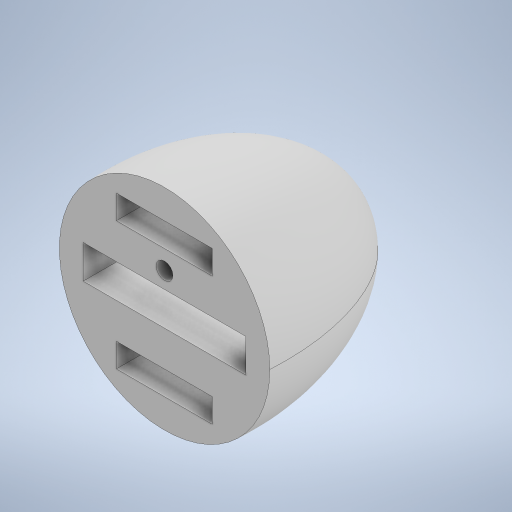
# Autodesk Inventor part: Bead Round Top copy 1
Saved by Autodesk Inventor 2024 (Build 280153000, 153)
## iProperties
Created: 2024-06-20
Part Number: Bead Round Top copy 1
Material: Generic
Document SubType Name: Modeling
Designer: waiy
Density: 1 g/cm^3
Appearance: Default
Author: waiy
Autodesk Inventor part; units mm, degrees
ref_plane "YZ Plane" through (0, 0, 0) normal (1, 0, 0) x (0, 1, 0)
ref_plane "XZ Plane" through (0, 0, 0) normal (0, 1, 0) x (-1, 0, 0)
ref_plane "XY Plane" through (0, 0, 0) normal (0, 0, 1) x (1, 0, 0)
sketch "Sketch1" plane through (0, 0, 0) normal (0, 1, 0) x (-1, 0, 0)
  ellipse E0 centre (0, 0) end of major axis (0, 17.78) minor radius 11.2075
  line L0 (11.1609, 1.6196) -> (-11.1609, 1.6196)
  line L1 (0, -17.78) -> (0, 1.6196)
  line L2 (8.595, 11.4106) -> (-8.6719, 11.4106)
  dimension "d0" = 17.78
  dimension "d11" = 9.7909
  constraints: 6 end point, 2 horizontal, 1 coincident, 1 midpoint, 6 other
  measures "d11" distance between parallel lines of L2 L0
revolve "Revolution1" add sketch "Sketch1" angle 360 about axis through (0, 0, -17.78) along (0, 0, 1) picked at (-2.3015, -10.0552) contours L0 L1 E0
sketch "Sketch2" plane through (0, 0, 1.6196) normal (0, 0, 1) x (1, 0, 0)
  line L0 (-8.636, 1.778) -> (8.636, 1.778)
  line L1 (8.636, 1.778) -> (8.636, -1.778)
  line L2 (8.636, -1.778) -> (-8.636, -1.778)
  line L3 (-8.636, -1.778) -> (-8.636, 1.778)
  line L4 (-8.636, 1.778) -> (8.636, -1.778) construction
  line L5 (8.636, 1.778) -> (-8.636, -1.778) construction
  point P0 (0, 0)
  dimension "d2" = 17.272
  dimension "d3" = 3.556
  constraints: 12 end point, 2 midpoint, 2 parallel, 1 horizontal, 1 perpendicular
  measures "d2" distance of L1.end L2.end
  measures "d3" distance of L0.end L1.end
extrude "Extrusion1" cut sketch "Sketch2" against normal blind 10.16
sketch "Sketch3" plane through (0, 0, 1.6196) normal (0, 0, 1) x (1, 0, 0)
  line L0 (-5.11, 8.0772) -> (5.05, 8.0772)
  line L1 (5.05, 8.0772) -> (5.05, 5.5372)
  line L2 (5.05, 5.5372) -> (-5.11, 5.5372)
  line L3 (-5.11, 5.5372) -> (-5.11, 8.0772)
  line L4 (-5.11, 8.0772) -> (5.05, 5.5372) construction
  line L5 (5.05, 8.0772) -> (-5.11, 5.5372) construction
  circle A0 centre (0, 0) radius 11.1609 projected
  line L6 (-11.1609, 0) -> (11.1609, 0)
  line L7 (11.2075, 0) -> (0, 0) projected
  line L8 (-5.11, -8.0772) -> (5.05, -8.0772)
  line L9 (5.05, -8.0772) -> (5.05, -5.5372)
  line L10 (5.05, -5.5372) -> (-5.11, -5.5372)
  line L11 (-5.11, -5.5372) -> (-5.11, -8.0772)
  point P0 (-0.03, 6.8072)
  dimension "d6" = 10.16
  dimension "d7" = 2.54
  dimension "d12" = 6.8072
  constraints: 22 end point, 4 symmetric about line, 2 midpoint, 2 parallel, 1 collinear, 1 horizontal, 1 perpendicular, 1 point on circle
  measures "d6" distance of L1.end L2.end
  measures "d7" distance of L0.end L1.end
  measures "d12" vertical distance of point (-0.03, 6.807) A0.centre
extrude "Extrusion2" cut sketch "Sketch3" against normal blind 7.62 contours L0 L1 L2 L3 | L11 L10 L9 L8
sketch "Sketch4" plane through (0, 0, 1.6196) normal (0, 0, 1) x (1, 0, 0)
  circle A0 centre (0, 3.497) radius 0.889
  point P0 (0, 0)
  dimension "d13" = 1.778
  constraints: 1 centre point
  measures "d13" diameter of A0
extrude "Extrusion3" cut sketch "Sketch4" against normal through all
body "Solid1"
